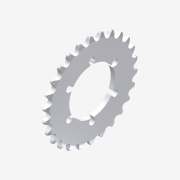
# Autodesk Inventor part: DriveTrain_Sprocket_S35-26-LE_AndyMark_am-0737
Saved by Autodesk Inventor 2012 (Build 160160000, 160)
## iProperties
Created: 2011-01-10
Part Number: DriveTrain_Sprocket_S35-26-LE_AndyMark_am-0737
Material: Aluminum-6061
Document SubType Name: Modeling
Designer: Autodesk Inc.
Density: 2.71 g/cm^3
Catalog Web Link: http://www.andymark.com/ProductDetails.asp?ProductCode=am%2D0737
Description: 26 tooth, 35 series aluminum sprocket for ANSI Roller Chain.
Vendor: Andy Mark Inc.
Mass: 35.0779 g
Surface Area: 87.5631 cm^2
Volume: 12.9439 cm^3
CustomPartVersion: 1
Category: Drive Train
Company: Autodesk Inc.
Author: Autodesk Inc.
Autodesk Inventor part; units mm, degrees
ref_plane "YZ Plane" through (0, 0, 0) normal (1, 0, 0) x (0, 1, 0)
ref_plane "XZ Plane" through (0, 0, 0) normal (0, 1, 0) x (-1, 0, 0)
sketch "Theoretical Tooth Profile" plane through (0, 0, 0) normal (0, 0, 1) x (1, 0, 0)
  circle A0 centre (0, 0) radius 39.5108 construction
  line L0 (0, 0) -> (0, 39.5108) construction
  line L1 (0, 0) -> (9.4556, 38.3627) construction
  circle A1 centre (0, 0) radius 42.0802
  arc A2 (-2.0607, 37.9405) -> (2.0607, 37.9405) centre (0, 39.5108) ccw
  line L2 (0, 39.5108) -> (9.4556, 38.3627) construction
  line L3 (0, 39.5108) -> (3.2325, 41.974) construction
  line L4 (3.2325, 41.974) -> (-2.9609, 39.5391) construction
  arc A3 (4.4267, 41.8467) -> (3.2081, 40.1679) centre (7.0601, 38.6535) ccw
  arc A4 (-3.2081, 40.1679) -> (-4.4267, 41.8467) centre (-7.0601, 38.6535) ccw
  line L5 (-7.0601, 38.6535) -> (-3.2081, 40.1679) construction
  arc A5 (-2.9609, 39.5391) -> (-2.0607, 37.9405) centre (3.2325, 41.974) ccw
  line L6 (-2.9609, 39.5391) -> (-3.2081, 40.1679)
  arc A6 (2.0607, 37.9405) -> (2.9609, 39.5391) centre (-3.2325, 41.974) ccw
  line L7 (3.2081, 40.1679) -> (2.9609, 39.5391)
  line L8 (0, 0) -> (5.0722, 41.7734) construction
  point P0 (4.7278, 38.9367)
  dimension "d0" = 79.0216
  dimension "d2" = 13.846
  dimension "d3" = 2.5908
  dimension "d10" = 127.308
  dimension "d11" = 15.846
  dimension "d12" = 4.064
  dimension "d13" = 6.6548
  dimension "d14" = 7.112
  dimension "d23" = 2.8575
  constraints: 18 end point, 15 point on circle, 7 centre point, 3 coincident, 3 point on line, 3 symmetric about line, 3 tangent, 1 equal radius, 1 midpoint, 1 parallel, 1 vertical, 1 other
  measures "d0" diameter of A0
  measures "d2" angle of L1 L0
  measures "d3" radius of A2
  measures "d10" angle of L3 L0
  measures "d11" angle of L4 L3
  measures "d12" distance of L2.start L3.end
  measures "d13" distance of L3.end L4.end
  measures "d14" distance of A3.centre L0.end
  measures "d23" distance from line of L8.end L2
sketch "Tooth Profile" plane through (0, 0, 0) normal (0, 0, 1) x (1, 0, 0)
  circle A0 centre (0, 0) radius 42.0802 projected
  line L0 (0, 0) -> (0, 39.5108) construction
  line L1 (0, 39.5108) -> (2.4067, 38.5516) construction
  arc A1 (-2.4067, 38.5516) -> (2.4067, 38.5516) centre (0, 39.5108) ccw
  line L2 (-2.4067, 38.5516) -> (0, 39.5108) construction
  arc A2 (-2.4067, 38.5516) -> (-4.1768, 41.8724) centre (-18.2625, 32.2319) ccw
  arc A3 (4.1768, 41.8724) -> (2.4067, 38.5516) centre (18.2625, 32.2319) ccw
  dimension "d44" = 136.538
  dimension "d45" = 2.5908
  dimension "d46" = 17.0688
  constraints: 8 point on circle, 7 end point, 3 centre point, 2 tangent, 1 coincident, 1 equal radius, 1 symmetric about line, 1 vertical
  measures "d44" angle of L1 L2
  measures "d45" radius of A1
  measures "d46" radius of A3
sketch "Section Profile" plane through (0, 0, 0) normal (1, 0, 0) x (0, 1, 0)
  line L0 (42.0802, 0) -> (-42.0802, 0) projected
  line L1 (33.6982, 1.9812) -> (-33.6982, 1.9812)
  line L2 (-33.6982, 1.9812) -> (-33.6982, -1.9812)
  line L3 (-33.6982, -1.9812) -> (33.6982, -1.9812)
  line L4 (33.6982, -1.9812) -> (33.6982, 1.9812)
  line L5 (33.6982, 1.9812) -> (42.0802, 1.9812) construction
  line L6 (42.0802, 1.9812) -> (42.0802, -1.9812) construction
  line L7 (42.0802, -1.9812) -> (33.6982, -1.9812) construction
  line L8 (33.6982, -1.9812) -> (33.6982, 1.9812)
  arc A0 (42.0802, 0.7906) -> (37.3165, 1.9812) centre (37.3165, -8.1439) ccw
  arc A1 (37.3165, -1.9812) -> (42.0802, -0.7906) centre (37.3165, 8.1439) ccw
  line L9 (37.3165, 1.9812) -> (0, 1.9812)
  line L10 (0, 1.9812) -> (0, -1.9812)
  line L11 (0, -1.9812) -> (37.3165, -1.9812)
  line L12 (0, 1.9812) -> (0, -1.9812)
  line L13 (42.0802, 0.7906) -> (42.0802, -0.7906)
  point P0 (0, 0)
  point P1 (0, 0)
  dimension "d30" = 3.9624
  dimension "d31" = 67.3964
  dimension "d32" = 3.9624
  dimension "d33" = 1.1906
  dimension "d34" = 10.1251
  dimension "d43" = 1.9812
  constraints: 26 end point, 7 midpoint, 5 perpendicular, 4 parallel, 4 point on circle, 3 point on line, 3 symmetric about line, 2 centre point, 2 horizontal, 2 tangent, 1 collinear, 1 other
  measures "d30" distance between parallel lines of L7 L5
  measures "d31" distance between parallel lines of L2 L4
  measures "d32" distance between parallel lines of L3 L1
  measures "d33" distance from line of L13.start L5
  measures "d34" radius of A0
  measures "d43" distance between parallel lines of L3 L0
revolve "Shroud" add sketch "Section Profile" angle 360 about axis through (0, 0, 1.9812) along (0, 0, -1) contours L10 L3 L2 L0 | L0 L2 L1 L10
revolve "Strand" add sketch "Section Profile" angle 360 about axis through (0, 0, 1.9812) along (0, 0, -1) contours L13 A1 L11 L4 L0 | L0 L4 L9 A0 L13 | L4 L3 L10 L0 | L0 L10 L1 L4
pattern_of_one "Strand Pattern"
extrude "Theoretical Tooth" cut sketch "Theoretical Tooth Profile" along normal through all both and the other way through all contours A3 L7 A6 A2 A5 L6 A4 A1 picked at (0.4927, 39.648)
extrude "Tooth" [suppressed]
pattern_circular "Tooth Pattern" count 26 over 360 about axis through (0, 0, -10) along (0, 0, 1) of "Theoretical Tooth"
ref_plane "Timing Plane" through (0, 39.5108, 0) normal (1, 0, 0) x (0, 1, 0)
sketch "Sketch4" plane through (0, 39.5108, 1.9812) normal (0, 0, 1) x (1, 0, 0)
  arc A0 (7.6251, -2.9816) -> (1.3385, -2.2183) centre (0, -39.5108) ccw projected
hole "Hole1" at (0, 0, 1.9812) direction (0, 0, -1) diameter 41.275 end through all
sketch "Sketch5" plane through (0, 39.5108, 1.9812) normal (0, 0, 1) x (1, 0, 0)
  arc A0 (16.1455, -5.8679) -> (10.2243, -3.6222) centre (0, -39.5108) ccw projected
  circle A1 centre (0, -39.5108) radius 23.8125
  point P0 (-23.8125, -39.5108)
  dimension "d58" = 47.625
  constraints: 2 horizontal alignment, 1 coincident, 2 other
hole "Hole2" at (-23.8125, 0, 1.9812) direction (0, 0, -1) diameter 5.2324 end through all
sketch "Sketch6" plane through (0, 39.5108, 1.9812) normal (0, 0, 1) x (1, 0, 0)
  circle A0 centre (-23.8125, -39.5108) radius 2.6162 projected
  circle A1 centre (-23.8125, -39.5108) radius 2.6162 projected
  circle A2 centre (0, -39.5108) radius 20.6375 projected
  arc A3 (7.6251, -2.9816) -> (10.2243, -3.6222) centre (9.4556, -1.1481) ccw projected
  arc A4 (7.6251, -2.9816) -> (1.3385, -2.2183) centre (0, -39.5108) ccw projected
  arc A5 (-1.3385, -2.2183) -> (1.3385, -2.2183) centre (0, 0) ccw projected
  arc A6 (-1.3385, -2.2183) -> (-7.6251, -2.9816) centre (0, -39.5108) ccw projected
  arc A7 (-10.2243, -3.6222) -> (-7.6251, -2.9816) centre (-9.4556, -1.1481) ccw projected
  arc A8 (-10.2243, -3.6222) -> (-16.1455, -5.8679) centre (0, -39.5108) ccw projected
  arc A9 (-18.5158, -7.1119) -> (-16.1455, -5.8679) centre (-18.3616, -4.5257) ccw projected
  arc A10 (-18.5158, -7.1119) -> (-23.7277, -10.7094) centre (0, -39.5108) ccw projected
  arc A11 (-25.7314, -12.4845) -> (-23.7277, -10.7094) centre (-26.2005, -9.9365) ccw projected
  arc A12 (-25.7314, -12.4845) -> (-29.9308, -17.2247) centre (0, -39.5108) ccw projected
  arc A13 (-31.4515, -19.4278) -> (-29.9308, -17.2247) centre (-32.5167, -17.0661) ccw projected
  arc A14 (-31.4515, -19.4278) -> (-34.3945, -25.0352) centre (0, -39.5108) ccw projected
  arc A15 (-35.3437, -27.5382) -> (-34.3945, -25.0352) centre (-36.9432, -25.5001) ccw projected
  arc A16 (-35.3437, -27.5382) -> (-36.8593, -33.687) centre (0, -39.5108) ccw projected
  arc A17 (-37.1819, -36.3444) -> (-36.8593, -33.687) centre (-39.2227, -34.7483) ccw projected
  arc A18 (-37.1819, -36.3444) -> (-37.1819, -42.6772) centre (0, -39.5108) ccw projected
  arc A19 (-36.8593, -45.3346) -> (-37.1819, -42.6772) centre (-39.2227, -44.2733) ccw projected
  arc A20 (-36.8593, -45.3346) -> (-35.3437, -51.4834) centre (0, -39.5108) ccw projected
  arc A21 (-34.3945, -53.9864) -> (-35.3437, -51.4834) centre (-36.9432, -53.5215) ccw projected
  arc A22 (-34.3945, -53.9864) -> (-31.4515, -59.5938) centre (0, -39.5108) ccw projected
  arc A23 (-29.9308, -61.7969) -> (-31.4515, -59.5938) centre (-32.5167, -61.9555) ccw projected
  arc A24 (-29.9308, -61.7969) -> (-25.7314, -66.5371) centre (0, -39.5108) ccw projected
  arc A25 (-23.7277, -68.3122) -> (-25.7314, -66.5371) centre (-26.2005, -69.085) ccw projected
  arc A26 (-23.7277, -68.3122) -> (-18.5158, -71.9097) centre (0, -39.5108) ccw projected
  arc A27 (-16.1455, -73.1537) -> (-18.5158, -71.9097) centre (-18.3616, -74.4959) ccw projected
  arc A28 (-16.1455, -73.1537) -> (-10.2243, -75.3993) centre (0, -39.5108) ccw projected
  arc A29 (-7.6251, -76.04) -> (-10.2243, -75.3993) centre (-9.4556, -77.8735) ccw projected
  arc A30 (-7.6251, -76.04) -> (-1.3385, -76.8033) centre (0, -39.5108) ccw projected
  arc A31 (1.3385, -76.8033) -> (-1.3385, -76.8033) centre (0, -79.0216) ccw projected
  arc A32 (1.3385, -76.8033) -> (7.6251, -76.04) centre (0, -39.5108) ccw projected
  arc A33 (10.2243, -75.3993) -> (7.6251, -76.04) centre (9.4556, -77.8735) ccw projected
  arc A34 (10.2243, -75.3993) -> (16.1455, -73.1537) centre (0, -39.5108) ccw projected
  arc A35 (18.5158, -71.9097) -> (16.1455, -73.1537) centre (18.3616, -74.4959) ccw projected
  arc A36 (18.5158, -71.9097) -> (23.7277, -68.3122) centre (0, -39.5108) ccw projected
  arc A37 (25.7314, -66.5371) -> (23.7277, -68.3122) centre (26.2005, -69.085) ccw projected
  arc A38 (25.7314, -66.5371) -> (29.9308, -61.7969) centre (0, -39.5108) ccw projected
  arc A39 (31.4515, -59.5938) -> (29.9308, -61.7969) centre (32.5167, -61.9555) ccw projected
  arc A40 (31.4515, -59.5938) -> (34.3945, -53.9864) centre (0, -39.5108) ccw projected
  arc A41 (35.3437, -51.4834) -> (34.3945, -53.9864) centre (36.9432, -53.5215) ccw projected
  arc A42 (35.3437, -51.4834) -> (36.8593, -45.3346) centre (0, -39.5108) ccw projected
  arc A43 (37.1819, -42.6772) -> (36.8593, -45.3346) centre (39.2227, -44.2733) ccw projected
  arc A44 (37.1819, -42.6772) -> (37.1819, -36.3444) centre (0, -39.5108) ccw projected
  arc A45 (36.8593, -33.687) -> (37.1819, -36.3444) centre (39.2227, -34.7483) ccw projected
  arc A46 (36.8593, -33.687) -> (35.3437, -27.5382) centre (0, -39.5108) ccw projected
  arc A47 (34.3945, -25.0352) -> (35.3437, -27.5382) centre (36.9432, -25.5001) ccw projected
  arc A48 (34.3945, -25.0352) -> (31.4515, -19.4278) centre (0, -39.5108) ccw projected
  arc A49 (29.9308, -17.2247) -> (31.4515, -19.4278) centre (32.5167, -17.0661) ccw projected
  arc A50 (29.9308, -17.2247) -> (25.7314, -12.4845) centre (0, -39.5108) ccw projected
  arc A51 (23.7277, -10.7094) -> (25.7314, -12.4845) centre (26.2005, -9.9365) ccw projected
  arc A52 (23.7277, -10.7094) -> (18.5158, -7.1119) centre (0, -39.5108) ccw projected
  arc A53 (16.1455, -5.8679) -> (18.5158, -7.1119) centre (18.3616, -4.5257) ccw projected
  arc A54 (16.1455, -5.8679) -> (10.2243, -3.6222) centre (0, -39.5108) ccw projected
  line L0 (-21.733, -41.0983) -> (-20.5764, -41.0983)
  line L1 (-21.733, -37.9233) -> (-20.5764, -37.9233)
  dimension "d69" = 3.175
  dimension "d70" = 1.5875
  constraints: 4 end point, 4 point on circle, 2 horizontal
  measures "d69" distance between parallel lines of L1 L0
  measures "d70" distance from line of A0.centre L0
extrude "Extrusion4" cut sketch "Sketch6" against normal up to next contours A0 L1 A2 L0
fillet "Fillet2" radius 0.3969 4 edges at (-21.733, 1.5875, 0) (-21.733, -1.5875, 0) (-20.5764, -1.5875, 0) (-20.5764, 1.5875, 0)
pattern_circular "Circular Pattern4" count 6 over 360 about axis through (0, 0, -116.7762) along (0, 0, 1) of "Hole2", "Extrusion4", "Fillet2"
equation "\"d3\" = 0.5 * da_Dr + da_SC"
equation "\"d12\" = 0.8 * da_Dr"
equation "\"d13\" = 1.3 * da_Dr + da_SC"
equation "\"d14\" = 1.4 * da_Dr"
equation "\"d23\" = da_Ha"
equation "\"d44\" = da_Alfa"
equation "\"d45\" = da_Ri"
equation "\"d46\" = da_Re"
equation "\"d30\" = da_Bf"
equation "\"d31\" = da_Ds"
equation "\"d32\" = d30"
equation "\"d33\" = da_Ba"
equation "\"d34\" = da_Rx"
equation "\"d43\" = 0.5 * d30"
equation "\"d40\" = da_pt"
equation "\"form_type\" = 0"
equation "\"da_p\" = 9.525"
equation "\"da_Dr\" = 5.08"
equation "\"da_SC\" = 0.0508"
equation "\"da_Ha\" = 2.8575"
equation "\"da_pt\" = 10.1346"
equation "\"da_Bf\" = 3.9624"
equation "\"da_Ba\" = 1.19063"
equation "\"da_Rx\" = 10.12508"
equation "\"da_Ra\" = 0.381"
equation "\"da_Bs\" = 4.59334"
equation "\"da_Ds\" = 67.39643"
equation "\"da_Re\" = 17.0688"
equation "\"da_Ri\" = 2.5908"
equation "\"da_Alfa\" = 136.538deg"
body "Solid1"
